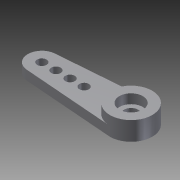
# Autodesk Inventor part: Horn
Saved by Autodesk Inventor 2012 (Build 160160000, 160)
## iProperties
Created: 2011-11-12
Part Number: Horn
Material: Default
Document SubType Name: Modeling
Designer: teguh
Density: 1 g/cm^3
Author: teguh
Autodesk Inventor part; units mm, degrees
ref_plane "YZ Plane" through (0, 0, 0) normal (1, 0, 0) x (0, 1, 0)
ref_plane "XZ Plane" through (0, 0, 0) normal (0, 1, 0) x (-1, 0, 0)
ref_plane "XY Plane" through (0, 0, 0) normal (0, 0, 1) x (1, 0, 0)
sketch "Sketch1" plane through (0, 0, 0) normal (0, 0, 1) x (1, 0, 0)
  circle A0 centre (-19, 0) radius 1
  circle A1 centre (-16, 0) radius 1
  circle A2 centre (-13, 0) radius 1
  circle A3 centre (-10, 0) radius 1
  circle A4 centre (0, 0) radius 1.5
  arc A5 (-19.2347, 2.9908) -> (-19.2347, -2.9908) centre (-19, 0) ccw
  arc A6 (-0.7018, -4.4449) -> (-0.7018, 4.4449) centre (0, 0) ccw
  line L0 (0, -4.5) -> (-19.2347, -2.9908)
  line L1 (0, 4.5) -> (-19.2347, 2.9908)
  dimension "d3" = 2
  dimension "d7" = 2
  dimension "d8" = 2
  dimension "d25" = 3
  dimension "d29" = 2
  dimension "d30" = 3
  dimension "d33" = 3
  dimension "d47" = 10
  dimension "d50" = 6
  dimension "d51" = 9
  dimension "d52" = 3
  constraints: 7 centre point, 6 point on circle, 4 end point, 2 coincident, 2 point on line, 2 tangent
  measures "d3" diameter of A0
  measures "d7" diameter of A1
  measures "d8" diameter of A2
  measures "d25" distance of A2.centre A1.centre
  measures "d29" diameter of A3
  measures "d30" distance of A3.centre A2.centre
  measures "d33" diameter of A4
  measures "d47" distance of point (0, 0) A3.centre
  measures "d50" diameter of A5
  measures "d51" diameter of A6
  measures "d52" distance of A1.centre A5.centre
extrude "Extrusion9" add sketch "Sketch1" along normal blind 2 contours L1 A6 L0 A5
sketch "Sketch8" plane through (0, 0, 2) normal (0, 0, 1) x (1, 0, 0)
  circle A0 centre (0, 0) radius 1.5 projected
  arc A1 (0, -4.5) -> (0, 4.5) centre (0, 0) ccw projected
  circle A2 centre (0, 0) radius 4.5
  dimension "d55" = 9
  constraints: 1 centre point, 1 coincident
  measures "d55" diameter of A2
extrude "Extrusion10" add sketch "Sketch8" along normal blind 2
sketch "Sketch9" plane through (0, 0, 4) normal (0, 0, 1) x (1, 0, 0)
  circle A0 centre (0, 0) radius 1.5 projected
  circle A1 centre (0, 0) radius 4.5 projected
  circle A2 centre (0, 0) radius 2.5
  dimension "d58" = 5
  constraints: 1 centre point, 1 coincident
  measures "d58" diameter of A2
hole "Hole2" at (0, 0, 4) direction (0, 0, -1) diameter 5 depth 2
body "Solid3"
